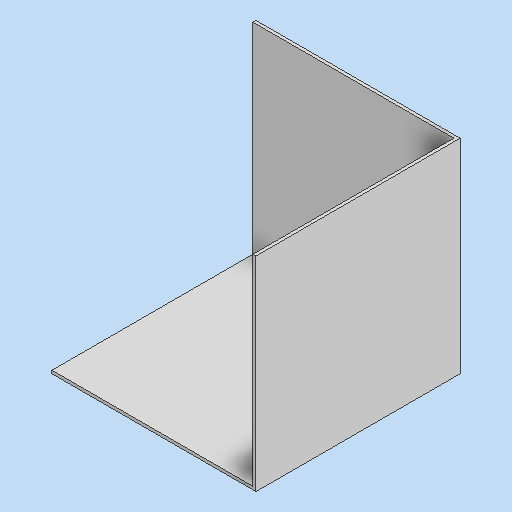
# Autodesk Inventor part: Chassis Constraints
Saved by Autodesk Inventor 2026 (Build 300175000, 175)
## iProperties
Created: 2026-01-28
Part Number: Chassis Constraints
Material: Generic
Document SubType Name: Modeling
Designer: mones
Density: 1 g/cm^3
Appearance: Default
Author: mones
Autodesk Inventor part; units mm, degrees
ref_plane "YZ Plane" through (0, 0, 0) normal (1, 0, 0) x (0, 1, 0)
ref_plane "XZ Plane" through (0, 0, 0) normal (0, 1, 0) x (-1, 0, 0)
ref_plane "XY Plane" through (0, 0, 0) normal (0, 0, 1) x (1, 0, 0)
sketch "Sketch1" plane through (0, 0, 0) normal (0, 1, 0) x (-1, 0, 0)
  line L0 (100, 100) -> (100, -100)
  line L1 (100, -100) -> (-100, -100)
  line L2 (-100, -100) -> (-100, 100)
  line L3 (-100, 100) -> (100, 100)
  line L4 (100, 100) -> (-100, -100) construction
  line L5 (100, -100) -> (-100, 100) construction
  point P0 (0, 0)
  dimension "d0" = 200
  dimension "d1" = 200
  constraints: 12 end point, 2 midpoint, 2 parallel, 1 perpendicular, 1 vertical
  measures "d0" distance of L0.start L0.end
  measures "d1" distance of L0.end L1.end
extrude "Extrusion1" add sketch "Sketch1" along normal blind 3
sketch "Sketch3" plane through (0, 3, 0) normal (0, 1, 0) x (1, 0, 0)
  line L0 (100, -100) -> (100, 100) projected
  line L1 (100, 100) -> (100, -100)
  line L2 (100, -100) -> (97, -100)
  line L3 (97, -100) -> (97, 100)
  line L4 (97, 100) -> (100, 100)
  dimension "d4" = 3
  constraints: 8 end point, 3 equal length, 1 perpendicular
  measures "d4" distance of L0.start L2.end
extrude "Extrusion2" add sketch "Sketch3" along normal blind 197
sketch "Sketch4" plane through (0, 3, 0) normal (0, 1, 0) x (1, 0, 0)
  line L0 (-100, 100) -> (97, 100)
  line L1 (97, 100) -> (97, 97)
  line L2 (97, 97) -> (-100, 97)
  line L3 (-100, 97) -> (-100, 100)
  dimension "d7" = 3
  constraints: 8 end point, 2 parallel, 1 horizontal, 1 perpendicular
  measures "d7" distance of L0.end L1.end
extrude "Extrusion3" add sketch "Sketch4" along normal blind 197
body "Solid1"
